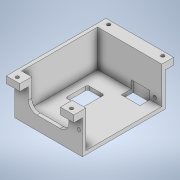
# Autodesk Inventor part: encaixe1 mouse
Saved by Autodesk Inventor 2022 (Build 260153000, 153)
## iProperties
Created: 2024-03-11
Part Number: encaixe1 mouse
Material: Generic
Document SubType Name: Modeling
Designer: admin
Density: 1 g/cm^3
Appearance: Default
Author: admin
Autodesk Inventor part; units mm, degrees
ref_plane "YZ Plane" through (0, 0, 0) normal (1, 0, 0) x (0, 1, 0)
ref_plane "XZ Plane" through (0, 0, 0) normal (0, 1, 0) x (-1, 0, 0)
ref_plane "XY Plane" through (0, 0, 0) normal (0, 0, 1) x (1, 0, 0)
sketch "Sketch1" plane through (0, 0, 0) normal (0, 1, 0) x (-1, 0, 0)
  line L0 (0, 0) -> (40, 0)
  line L1 (40, 0) -> (40, -49)
  line L2 (40, -49) -> (0, -49)
  line L3 (0, -49) -> (0, 0)
  dimension "d0" = 40
  dimension "d1" = 49
  constraints: 8 end point, 2 parallel, 1 horizontal, 1 perpendicular
  measures "d0" distance of L1.end L2.end
  measures "d1" distance of L0.end L1.end
extrude "Extrusion1" add sketch "Sketch1" along normal blind 24
sketch "Sketch2" plane through (0, 24, 0) normal (0, 1, 0) x (1, 0, 0)
  line L0 (0, 0) -> (0, 49) projected
  line L1 (0, 49) -> (-40, 49) projected
  line L2 (0, 0) -> (-2, 0)
  line L3 (-2, 0) -> (-2, 49)
  line L4 (-2, 49) -> (0, 49)
  line L5 (0, 49) -> (0, 0)
  line L6 (-40, 49) -> (-40, 0) projected
  line L7 (-40, 0) -> (-38, 0)
  line L8 (-38, 0) -> (-38, 49)
  line L9 (-38, 49) -> (-40, 49)
  line L10 (-40, 49) -> (-40, 0)
  line L11 (0, 0) -> (-40, 0)
  line L12 (-40, 0) -> (-40, 2)
  line L13 (-40, 2) -> (0, 2)
  line L14 (0, 2) -> (0, 0)
  line L15 (0, 49) -> (-40, 49)
  line L16 (-40, 49) -> (-40, 47)
  line L17 (-40, 47) -> (0, 47)
  line L18 (0, 47) -> (0, 49)
  line L19 (-2, 47) -> (-38, 47)
  line L20 (-38, 47) -> (-38, 2)
  line L21 (-38, 2) -> (-2, 2)
  line L22 (-2, 2) -> (-2, 47)
  point P0 (-38, 47)
  dimension "d4" = 2
  dimension "d5" = 2
  dimension "d6" = 2
  dimension "d7" = 2
  constraints: 40 end point, 10 parallel, 8 point on line, 5 horizontal, 5 perpendicular
  measures "d4" distance of L3.end L4.end
  measures "d5" distance of L9.end L8.end
  measures "d6" distance of L11.end L12.end
  measures "d7" distance of L16.end L15.end
extrude "Extrusion2" cut sketch "Sketch2" against normal blind 21.75 contours L13 L8 L17 L3
sketch "Sketch3" plane through (-40, 0, 0) normal (0, 0, 1) x (1, 0, 0)
  line L0 (0, 24) -> (40, 24) projected
  line L1 (0, 0) -> (40, 0) projected
  line L2 (0, 24) -> (8, 24)
  line L3 (8, 24) -> (8, 0)
  line L4 (8, 0) -> (0, 0)
  line L5 (0, 0) -> (0, 24)
  line L6 (0, 0) -> (0, 24) projected
  line L7 (40, 0) -> (40, 24) projected
  line L8 (0, 0) -> (40, 0)
  line L9 (40, 0) -> (40, 8)
  line L10 (40, 8) -> (0, 8)
  line L11 (0, 8) -> (0, 0)
  line L12 (38, 24) -> (2, 24) projected
  line L13 (40, 0) -> (32, 0)
  line L14 (32, 0) -> (32, 24)
  line L15 (32, 24) -> (40, 24)
  line L16 (40, 24) -> (40, 0)
  line L17 (8, 24) -> (32, 24)
  line L18 (32, 24) -> (32, 8)
  line L19 (32, 8) -> (8, 8)
  line L20 (8, 8) -> (8, 24)
  point P0 (8, 8)
  dimension "d10" = 8
  dimension "d11" = 8
  dimension "d12" = 8
  constraints: 32 end point, 8 parallel, 5 point on line, 4 horizontal, 4 perpendicular
  measures "d10" distance of L3.end L4.end
  measures "d11" distance of L9.end L8.end
  measures "d12" distance of L14.end L15.end
extrude "Extrusion3" cut sketch "Sketch3" against normal blind 21 contours L0 L14 L10 L3
fillet "Fillet1" radius 5 2 edges at (-32, 8, -1) (-8, 8, -1)
sketch "Sketch4" plane through (-40, 0, 0) normal (0, 0, 1) x (1, 0, 0)
  line L0 (0, 0) -> (0, 24) projected
  line L1 (8, 13) -> (8, 24) projected
  line L2 (0, 24) -> (8, 24)
  line L3 (8, 24) -> (8, 20)
  line L4 (8, 20) -> (0, 20)
  line L5 (0, 20) -> (0, 24)
  line L6 (32, 24) -> (40, 24) projected
  line L7 (32, 13) -> (32, 24) projected
  line L8 (40, 24) -> (32, 24)
  line L9 (32, 24) -> (32, 20)
  line L10 (32, 20) -> (40, 20)
  line L11 (40, 20) -> (40, 24)
  point P0 (40, 0)
  point P1 (0, 20)
  dimension "d16" = 4
  dimension "d17" = 4
  constraints: 16 end point, 4 parallel, 2 horizontal, 2 perpendicular, 2 point on line
  measures "d16" distance of L2.end L3.end
  measures "d17" distance of L9.end L8.end
extrude "Extrusion4" add sketch "Sketch4" along normal blind 5
sketch "Sketch5" plane through (0, 0, -49) normal (0, 0, -1) x (-1, 0, 0)
  line L0 (40, 0) -> (40, 24) projected
  line L1 (0, 24) -> (40, 24)
  line L2 (40, 24) -> (40, 20)
  line L3 (40, 20) -> (0, 20)
  line L4 (0, 20) -> (0, 24)
  point P0 (0, 0)
  dimension "d20" = 4
  constraints: 8 end point, 2 parallel, 1 horizontal, 1 perpendicular, 1 point on line
  measures "d20" distance of L1.end L2.end
extrude "Extrusion5" add sketch "Sketch5" along normal blind 5
sketch "Sketch6" plane through (-2, 24, -47) normal (-1, 0, 0) x (0, 0, 1)
  line L0 (0, 0) -> (0, -21.75) projected
  line L1 (0, 0) -> (45, 0) projected
  line L2 (0, -21.75) -> (45, -21.75)
  line L3 (45, -21.75) -> (45, 0)
  line L4 (45, 0) -> (0, 0)
  line L5 (0, 0) -> (0, -21.75)
  point P0 (47, -24)
  constraints: 8 end point, 2 parallel, 1 horizontal, 1 perpendicular
extrude "Extrusion6" cut sketch "Sketch6" against normal blind 10
sketch "Sketch7" plane through (0, 2.25, 0) normal (0, 1, 0) x (1, 0, 0)
  line L0 (-38, 47) -> (-23, 47)
  line L1 (-23, 47) -> (-23, 36)
  line L2 (-23, 36) -> (-38, 36)
  line L3 (-38, 36) -> (-38, 47)
  line L4 (-23, 36) -> (-33, 36)
  line L5 (-33, 36) -> (-33, 23)
  line L6 (-33, 23) -> (-23, 23)
  line L7 (-23, 23) -> (-23, 36)
  line L8 (-38, 47) -> (0, 47) projected
  line L9 (-23, 23) -> (-18, 23)
  line L10 (-18, 23) -> (-18, 47)
  line L11 (-18, 47) -> (-23, 47)
  line L12 (-23, 47) -> (-23, 23)
  line L13 (-18, 47) -> (-7, 47)
  line L14 (-7, 47) -> (-7, 41)
  line L15 (-7, 41) -> (-18, 41)
  line L16 (-18, 41) -> (-18, 47)
  point P0 (0, 0)
  point P1 (-7, 47)
  dimension "d25" = 15
  dimension "d26" = 11
  dimension "d27" = 10
  dimension "d28" = 13
  dimension "d29" = 5
  dimension "d30" = 11
  dimension "d31" = 6
  constraints: 32 end point, 8 parallel, 4 horizontal, 4 perpendicular, 1 point on line
  measures "d25" distance of L1.end L2.end
  measures "d26" distance of L0.end L1.end
  measures "d27" distance of L6.end L5.end
  measures "d28" distance of L5.end L4.end
  measures "d29" distance of L11.end L10.end
  measures "d30" distance of L14.end L15.end
  measures "d31" distance of L13.end L14.end
extrude "Extrusion7" cut sketch "Sketch7" against normal blind 10 contours L7 L6 L5 L2 | L8 L14 L15 L10
sketch "Sketch8" plane through (-38, 24, -47) normal (0, 0, 1) x (1, 0, 0)
  line L0 (20, -24) -> (31, -24)
  line L1 (31, -24) -> (31, -17)
  line L2 (31, -17) -> (20, -17)
  line L3 (20, -17) -> (20, -24)
  point P0 (38, -24)
  dimension "d34" = 11
  dimension "d35" = 7
  constraints: 8 end point, 2 parallel, 1 horizontal, 1 perpendicular
  measures "d34" distance of L2.end L1.end
  measures "d35" distance of L1.end L0.end
extrude "Extrusion8" cut sketch "Sketch8" against normal blind 1
fillet "Fillet2" radius 1 4 edges at (-33, 1.125, -36) (-23, 1.125, -36) (-33, 1.125, -23) (-23, 1.125, -23)
sketch "Sketch9" plane through (-38, 24, -48) normal (0, 0, 1) x (1, 0, 0)
  line L0 (31, -24) -> (20, -24) projected
  line L1 (20, -17) -> (31, -17)
  line L2 (31, -17) -> (31, -24)
  line L3 (31, -24) -> (20, -24)
  line L4 (20, -24) -> (20, -17)
  line L5 (20, -24) -> (20, -17) projected
  line L6 (20, -17) -> (19, -17)
  line L7 (19, -17) -> (19, -24)
  line L8 (19, -24) -> (20, -24)
  line L9 (20, -24) -> (20, -17)
  line L10 (31, -17) -> (32, -17)
  line L11 (32, -17) -> (32, -24)
  line L12 (32, -24) -> (31, -24)
  line L13 (31, -24) -> (31, -17)
  point P0 (38, -24)
  point P1 (31, -24)
  dimension "d69" = 1
  dimension "d70" = 1
  constraints: 24 end point, 6 parallel, 3 horizontal, 3 perpendicular
  measures "d69" distance of L8.end L7.end
  measures "d70" distance of L11.end L12.end
extrude "Extrusion9" add sketch "Sketch9" against normal blind 1.5
sketch "Sketch10" plane through (0, 0, 0) normal (0, -1, 0) x (1, 0, 0)
  line L0 (-8, 5) -> (0, 5) projected
  line L1 (0, 5) -> (-4, 5)
  line L2 (-4, 5) -> (-4, 2.5)
  line L3 (-4, 2.5) -> (0, 2.5)
  line L4 (0, 2.5) -> (0, 5)
  circle A0 centre (-4, 2.5) radius 1
  line L5 (-40, 0) -> (-40, 5) projected
  line L6 (-40, 5) -> (-36, 5)
  line L7 (-36, 5) -> (-36, 2.5)
  line L8 (-36, 2.5) -> (-40, 2.5)
  line L9 (-40, 2.5) -> (-40, 5)
  circle A1 centre (-36, 2.5) radius 1
  line L10 (-40, 5) -> (-40, -54) projected
  line L11 (-40, -54) -> (-36, -54)
  line L12 (-36, -54) -> (-36, -51.5)
  line L13 (-36, -51.5) -> (-40, -51.5)
  line L14 (-40, -51.5) -> (-40, -54)
  circle A2 centre (-36, -51.5) radius 1
  line L15 (0, -54) -> (0, -47) projected
  line L16 (0, -54) -> (-4, -54)
  line L17 (-4, -54) -> (-4, -51.5)
  line L18 (-4, -51.5) -> (0, -51.5)
  line L19 (0, -51.5) -> (0, -54)
  circle A3 centre (-4, -51.5) radius 1
  point P0 (0, 0)
  dimension "d41" = 4
  dimension "d42" = 2.5
  dimension "d43" = 2
  dimension "d44" = 4
  dimension "d45" = 2.5
  dimension "d46" = 2
  dimension "d49" = 4
  dimension "d50" = 2.5
  dimension "d51" = 2
  dimension "d53" = 4
  dimension "d54" = 2.5
  dimension "d55" = 2
  constraints: 32 end point, 8 parallel, 4 centre point, 4 coincident, 4 horizontal, 4 perpendicular
  measures "d41" distance of L3.end L2.end
  measures "d42" distance of L2.end L1.end
  measures "d43" diameter of A0
  measures "d44" distance of L7.end L8.end
  measures "d45" distance of L6.end L7.end
  measures "d46" diameter of A1
  measures "d49" distance of L13.end L12.end
  measures "d50" distance of L12.end L11.end
  measures "d51" diameter of A2
  measures "d53" distance of L17.end L18.end
  measures "d54" distance of L16.end L17.end
  measures "d55" diameter of A3
extrude "Extrusion10" cut sketch "Sketch10" against normal blind 30 contours A0 L3 L2 | L2 L3 A0 | A1 L7 L8 | L8 L7 A1 | A2 L12 L13 | L13 L12 A2 | A3 L17 L18 | L18 L17 A3
sketch "Sketch11" plane through (-8, 20, 0) normal (0, -1, 0) x (1, 0, 0)
  circle A0 centre (4, 2.5) radius 1 projected
  circle A1 centre (4, 2.5) radius 2
  circle A2 centre (-28, 2.5) radius 1 projected
  circle A3 centre (-28, 2.5) radius 2
  circle A4 centre (4, -51.5) radius 1 projected
  circle A5 centre (4, -51.5) radius 2
  circle A6 centre (-28, -51.5) radius 1 projected
  circle A7 centre (-28, -51.5) radius 2
  point P0 (8, 0)
  dimension "d58" = 4
  dimension "d59" = 4
  dimension "d60" = 4
  dimension "d61" = 4
  constraints: 4 centre point, 4 coincident
  measures "d58" diameter of A1
  measures "d59" diameter of A3
  measures "d60" diameter of A5
  measures "d61" diameter of A7
extrude "Extrusion11" cut sketch "Sketch11" against normal blind 2 contours A1 | A2 | A3 | A4 | A5 | A6 | A7
sketch "Sketch12" plane through (-40, 0, 0) normal (0, 0, 1) x (1, 0, 0)
  line L0 (0, 20) -> (40, 20) projected
  line L1 (40, 20) -> (38, 20)
  line L2 (38, 20) -> (38, 13)
  line L3 (38, 13) -> (40, 13)
  line L4 (40, 13) -> (40, 20)
  circle A0 centre (38, 13) radius 1
  point P0 (40, 0)
  dimension "d64" = 2
  dimension "d65" = 7
  dimension "d66" = 2
  constraints: 8 end point, 2 parallel, 1 centre point, 1 coincident, 1 horizontal, 1 perpendicular
  measures "d64" distance of L3.end L2.end
  measures "d65" distance of L2.end L1.end
  measures "d66" diameter of A0
extrude "Extrusion12" cut sketch "Sketch12" against normal blind 5 contours A0 L3 L2 | L2 L3 A0
sketch "Sketch13" plane through (0, 20, -49) normal (0, 0, -1) x (-1, 0, 0)
  line L0 (6, -13) -> (19, -13) projected
  line L1 (6, -13) -> (4, -13)
  line L2 (4, -13) -> (4, -15)
  line L3 (4, -15) -> (6, -15)
  line L4 (6, -15) -> (6, -13)
  circle A0 centre (4, -15) radius 1
  point P0 (0, -20)
  dimension "d71" = 2
  dimension "d72" = 2
  dimension "d73" = 2
  constraints: 8 end point, 2 parallel, 1 centre point, 1 coincident, 1 horizontal, 1 perpendicular
  measures "d71" distance of L3.end L2.end
  measures "d72" distance of L2.end L1.end
  measures "d73" diameter of A0
extrude "Extrusion13" cut sketch "Sketch13" against normal blind 3 contours A0 L3 L2 | L2 L3 A0
body "Solid1"
